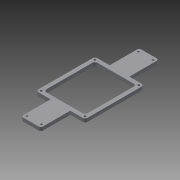
# Autodesk Inventor part: phone_plate
Saved by Autodesk Inventor 2015 (Build 190159000, 159)
## iProperties
Created: 2015-12-01
Part Number: phone_plate
Material: Generic
Document SubType Name: Modeling
Designer: jufranz
Density: 1 g/cm^3
Appearance: Default
Author: jufranz
Autodesk Inventor part; units mm, degrees
ref_plane "YZ Plane" through (0, 0, 0) normal (1, 0, 0) x (0, 1, 0)
ref_plane "XZ Plane" through (0, 0, 0) normal (0, 1, 0) x (-1, 0, 0)
ref_plane "XY Plane" through (0, 0, 0) normal (0, 0, 1) x (1, 0, 0)
sketch "Sketch1" plane through (0, 0, 0) normal (0, 1, 0) x (-1, 0, 0)
  line L0 (37.5, 45) -> (-37.5, 45)
  line L1 (-37.5, 45) -> (-37.5, -45)
  line L2 (-37.5, -45) -> (37.5, -45)
  line L3 (37.5, -45) -> (37.5, 45)
  point P0 (0, 0)
  point P1 (37.5, 0)
  point P2 (0, 45)
  dimension "d0" = 90
  dimension "d1" = 75
  constraints: 8 end point, 2 midpoint, 2 parallel, 1 horizontal, 1 horizontal alignment, 1 perpendicular, 1 vertical alignment
  measures "d0" distance of L2.end L0.start
  measures "d1" distance between parallel lines of L1 L3
extrude "Extrusion1" add sketch "Sketch1" along normal blind 5.334
sketch "Sketch2" plane through (0, 5.334, 0) normal (0, 1, 0) x (1, 0, 0)
  line L0 (-31.5, -39) -> (31.5, -39)
  line L1 (31.5, -39) -> (31.5, 39)
  line L2 (31.5, 39) -> (-31.5, 39)
  line L3 (-31.5, 39) -> (-31.5, -39)
  line L4 (-37.5, -45) -> (37.5, -45) projected
  line L5 (37.5, 45) -> (-37.5, 45) projected
  line L6 (-37.5, 45) -> (-37.5, -45) projected
  line L7 (37.5, -45) -> (37.5, 45) projected
  point P0 (0, 0)
  dimension "d4" = 6
  dimension "d5" = 6
  dimension "d6" = 6
  dimension "d7" = 6
  constraints: 8 end point, 2 parallel, 1 horizontal, 1 perpendicular
  measures "d4" distance between parallel lines of L4 L0
  measures "d5" distance between parallel lines of L5 L2
  measures "d6" distance between parallel lines of L6 L3
  measures "d7" distance between parallel lines of L7 L1
extrude "Extrusion2" cut sketch "Sketch2" against normal through all contours L3 L2 L1 L0
sketch "Sketch3" plane through (0, 5.334, 0) normal (0, 1, 0) x (1, 0, 0)
  line L0 (-37.5, -45) -> (37.5, -45) projected
  line L1 (-37.5, 45) -> (-37.5, -45) projected
  line L2 (37.5, -45) -> (37.5, 45) projected
  line L3 (37.5, 45) -> (-37.5, 45) projected
  point P0 (0, 0)
  point P1 (-33.5, -41)
  point P2 (-33.5, 41)
  point P3 (33.5, 41)
  point P4 (33.5, -41)
  dimension "d10" = 4
  dimension "d11" = 4
  dimension "d12" = 4
  dimension "d13" = 4
  constraints: 2 horizontal alignment, 2 vertical alignment
  measures "d10" distance from line of L0 point (-33.5, -41)
  measures "d11" distance from line of L1 point (-33.5, -41)
  measures "d12" distance from line of L2 point (33.5, 41)
  measures "d13" distance from line of L3 point (33.5, 41)
hole "Hole1" at (-33.5, 5.334, 41) at (-33.5, 5.334, -41) at (33.5, 5.334, -41) at (33.5, 5.334, 41) direction (0, -1, 0) diameter 3.2 end through all
fillet "Fillet1" radius 4 8 edges at (-37.5, 2.667, 45) (-31.5, 2.667, 39) (37.5, 2.667, 45) (37.5, 2.667, -45) (31.5, 2.667, -39) (31.5, 2.667, 39) (-31.5, 2.667, -39) (-37.5, 2.667, -45)
sketch "Sketch4" plane through (33.5, 0, -45) normal (0, 0, -1) x (-1, 0, 0)
  line L0 (6, 5.334) -> (61, 5.334) projected
  line L1 (61, 0) -> (6, 0) projected
  line L2 (48.5, 5.334) -> (18.5, 5.334)
  line L3 (18.5, 5.334) -> (18.5, 0)
  line L4 (18.5, 0) -> (48.5, 0)
  line L5 (48.5, 0) -> (48.5, 5.334)
  point P0 (33.5, 0)
  dimension "d22" = 30
  dimension "d23" = 15
  constraints: 8 end point, 2 parallel, 2 point on line, 1 horizontal, 1 perpendicular
  measures "d22" distance between parallel lines of L3 L5
  measures "d23" distance from line of L5 point (33.5, 0)
extrude "Extrusion3" add sketch "Sketch4" along normal blind 45
sketch "Sketch5" plane through (0, 5.334, 0) normal (0, 1, 0) x (1, 0, 0)
  line L0 (-15, 90) -> (15, 90) projected
  point P0 (0, 0)
  point P1 (-11, 85)
  point P2 (11, 85)
  dimension "d27" = 22
  dimension "d28" = 11
  dimension "d29" = 5
  constraints: 1 horizontal alignment
  measures "d27" distance of point (-11, 85) point (11, 85)
  measures "d28" horizontal distance of point (0, 0) point (11, 85)
  measures "d29" distance from line of L0 point (-11, 85)
hole "Hole2" at (-11, 5.334, -85) at (11, 5.334, -85) direction (0, -1, 0) diameter 3 end through all
mirror "Mirror1" about plane through (0, 0, 0) normal (0, 0, 1) of "Extrusion3", "Hole2"
equation "\"d5\" = d4"
equation "\"d6\" = d4"
equation "\"d7\" = d4"
equation "\"d11\" = d10"
equation "\"d12\" = d10"
equation "\"d13\" = d10"
equation "\"d23\" = 0.5 * d22"
equation "\"d28\" = 0.5 * d27"
body "Solid1"
